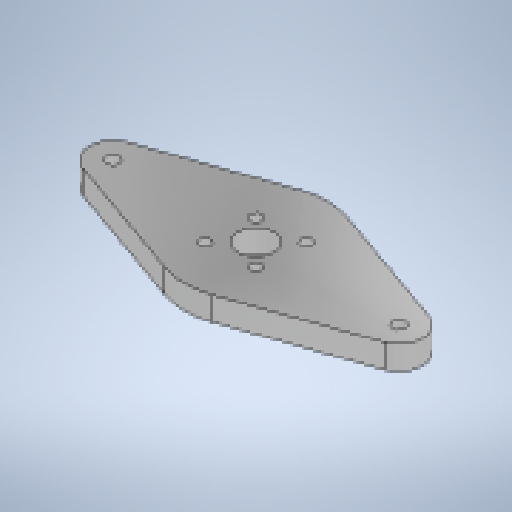
# Autodesk Inventor part: Upright - Top
Saved by Autodesk Inventor 2023.2 (Build 272271000, 271)
## iProperties
Created: 2023-10-16
Part Number: Upright - Top
Material: Aluminum 6061
Document SubType Name: Modeling
Designer: Nathan Cai
Mass: 35.1796 g
Surface Area: 59.484 cm^2
Volume: 13.0295 cm^3
Density: 2.7 g/cm^3
Appearance: Aluminum - Flat
Author: Nathan Cai
Autodesk Inventor part; units mm, degrees
ref_plane "YZ Plane" through (0, 0, 0) normal (1, 0, 0) x (0, 1, 0)
ref_plane "XZ Plane" through (0, 0, 0) normal (0, 1, 0) x (-1, 0, 0)
ref_plane "XY Plane" through (0, 0, 0) normal (0, 0, 1) x (1, 0, 0)
sketch "Sketch1" plane through (0, 0, 0) normal (0, 1, 0) x (-1, 0, 0)
  circle A0 centre (0, 0) radius 38.1 construction
  line L0 (38.1, 0) -> (0, 0) construction
  circle A1 centre (38.1, 0) radius 1.7526
  circle A2 centre (0, 0) radius 4.7625
  circle A3 centre (-38.1, 0) radius 1.7526
  circle A4 centre (0, 0) radius 9.5 construction
  circle A5 centre (0, 0) radius 8 construction
  line L1 (0, 0) -> (-6.7175, -6.7175) construction
  line L2 (0, 0) -> (6.7175, -6.7175) construction
  circle A6 centre (-5.6569, -5.6569) radius 1.5
  circle A7 centre (6.7175, -6.7175) radius 1.5
  circle A8 centre (-6.7175, 6.7175) radius 1.5
  circle A9 centre (5.6569, 5.6569) radius 1.5
  circle A10 centre (38.1, 0) radius 6.35
  circle A11 centre (-38.1, 0) radius 6.35
  circle A12 centre (0, 0) radius 19.05
  line L3 (40.2167, -5.9868) -> (6.35, -17.9605)
  line L4 (40.2167, 5.9868) -> (6.35, 17.9605)
  line L5 (-40.2167, -5.9868) -> (-6.35, -17.9605)
  line L6 (-40.2167, 5.9868) -> (-6.35, 17.9605)
  point P0 (-6.35, 17.9605)
  point P1 (-6.35, -17.9605)
  dimension "d0" = 76.2
  dimension "d8" = 16
  dimension "d16" = 12.7
  dimension "d21" = 38.1
  dimension "d1" = 3.5052
  dimension "d2" = 9.525
  dimension "d5" = 360
  dimension "d7" = 19
  dimension "d9" = 135
  dimension "d10" = 3
  dimension "d11" = 3
  dimension "d14" = 360
  dimension "d19" = 360
  dimension "d24" = 360
  constraints: 14 end point, 9 centre point, 8 coincident, 2 point on circle, 2 symmetric about line, 1 horizontal, 1 horizontal alignment, 1 perpendicular, 1 point on line, 45 other
  measures "d1" diameter of A1
  measures "d2" diameter of A2
  measures "d7" diameter of A4
  measures "d9" angle of L0 L1
  measures "d10" diameter of A6
  measures "d11" diameter of A7
extrude "Extrusion1" add sketch "Sketch1" along normal blind 6.35
body "Solid1"
